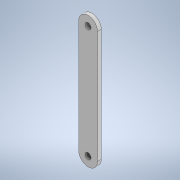
# Autodesk Inventor part: cięgno silnika platformy
Saved by Autodesk Inventor 2021 (Build 250183000, 183)
## iProperties
Created: 2022-04-11
Part Number: cięgno silnika platformy
Material: Generic
Document SubType Name: Modeling
Designer: Łukasz
Density: 1 g/cm^3
Appearance: Default
Author: Łukasz
Autodesk Inventor part; units mm, degrees
ref_plane "YZ Plane" through (0, 0, 0) normal (1, 0, 0) x (0, 1, 0)
ref_plane "XZ Plane" through (0, 0, 0) normal (0, 1, 0) x (-1, 0, 0)
ref_plane "XY Plane" through (0, 0, 0) normal (0, 0, 1) x (1, 0, 0)
sketch "Sketch1" plane through (0, 0, 0) normal (0, 0, 1) x (1, 0, 0)
  circle A0 centre (0, 0) radius 4
  circle A1 centre (0, 0) radius 12.5
  circle A2 centre (0, 150) radius 4
  circle A3 centre (0, 150) radius 12.5
  line L0 (-12.5, 150) -> (-12.5, 0)
  line L1 (12.5, 150) -> (12.5, 0)
  dimension "d0" = 8
  dimension "d1" = 25
  dimension "d2" = 8
  dimension "d3" = 25
  dimension "d4" = 150
  dimension "d5" = 0
  constraints: 4 centre point, 4 end point, 4 point on circle, 3 coincident, 2 tangent
  measures "d0" diameter of A0
  measures "d1" diameter of A1
  measures "d2" diameter of A2
  measures "d3" diameter of A3
  measures "d4" distance of A0.centre A2.centre
  measures "d5" horizontal distance of A0.centre A2.centre
extrude "Extrusion1" add sketch "Sketch1" along normal blind 5
equation "\"d2\" = d0"
equation "\"d3\" = d1"
body "Solid1"
